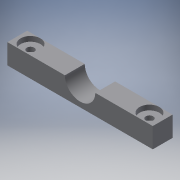
# Autodesk Inventor part: BaseOfSwallowWaterer
Saved by Autodesk Inventor 2019.3 (Build 233278000, 278)
## iProperties
Created: 2019-04-02
Part Number: BaseOfSwallowWaterer
Material: Generic
Document SubType Name: Modeling
Designer: steele
Density: 1 g/cm^3
Appearance: Default
Author: steele
Autodesk Inventor part; units mm, degrees
ref_plane "YZ Plane" through (0, 0, 0) normal (1, 0, 0) x (0, 1, 0)
ref_plane "XZ Plane" through (0, 0, 0) normal (0, 1, 0) x (-1, 0, 0)
ref_plane "XY Plane" through (0, 0, 0) normal (0, 0, 1) x (1, 0, 0)
sketch "Sketch1" plane through (0, 0, 0) normal (0, 1, 0) x (-1, 0, 0)
  line L0 (69.85, 9.525) -> (-69.85, 9.525)
  line L1 (-69.85, 9.525) -> (-69.85, -9.525)
  line L2 (-69.85, -9.525) -> (69.85, -9.525)
  line L3 (69.85, -9.525) -> (69.85, 9.525)
  line L4 (69.85, 9.525) -> (-69.85, -9.525) construction
  line L5 (-69.85, 9.525) -> (69.85, -9.525) construction
  point P0 (0, 0)
  dimension "d0" = 139.7
  dimension "d1" = 19.05
  constraints: 12 end point, 2 midpoint, 2 parallel, 1 horizontal, 1 perpendicular
  measures "d0" distance of L0.start L0.end
  measures "d1" distance of L2.end L0.start
extrude "Extrusion1" add sketch "Sketch1" along normal blind 19.3675
sketch "Sketch2" plane through (-69.85, 0, 9.525) normal (0, 0, 1) x (1, 0, 0)
  line L0 (0, 19.3675) -> (139.7, 19.3675) projected
  arc A0 (55.245, 19.3675) -> (84.455, 19.3675) centre (69.85, 19.3675) ccw
  point P0 (69.85, 0)
  dimension "d4" = 29.21
  constraints: 2 point on circle, 2 point on line, 1 centre point, 1 midpoint
  measures "d4" diameter of A0
extrude "Extrusion2" cut sketch "Sketch2" against normal through all
sketch "Sketch3" plane through (0, 19.3675, 0) normal (0, 1, 0) x (1, 0, 0)
  line L0 (-69.85, -9.525) -> (-14.605, -9.525) projected
  line L1 (-69.85, 9.525) -> (-69.85, -9.525) projected
  line L2 (-14.605, 9.525) -> (-69.85, 9.525) projected
  line L3 (69.85, -9.525) -> (69.85, 9.525) projected
  line L4 (69.85, 9.525) -> (14.605, 9.525) projected
  line L5 (14.605, -9.525) -> (69.85, -9.525) projected
  point P0 (0, 0)
  point P1 (-57.15, 0)
  point P2 (57.15, 0)
  dimension "d7" = 9.525
  dimension "d8" = 12.7
  dimension "d13" = 9.525
  dimension "d14" = 12.7
  measures "d7" distance from line of point (-57.15, 0) L0
  measures "d8" distance from line of L1 point (-57.15, 0)
  measures "d13" distance from line of point (57.15, 0) L5
  measures "d14" distance from line of point (57.15, 0) L3
hole "Hole1" at (-57.15, 19.3675, 0) at (57.15, 19.3675, 0) direction (0, -1, 0) diameter 7.1374 end through all clearance for "Hex Head Bolt" size "1/4" standard "Ansi Unified Screw Threads"
body "Solid1"
